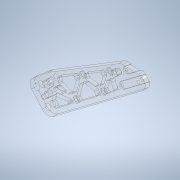
# Autodesk Inventor part: アーム アーム先端根本ポリカパーツ(ミラー)
Saved by Autodesk Inventor 2020.2 (Build 242310000, 310)
## iProperties
Created: 2020-05-02
Part Number: アーム アーム先端根本ポリカパーツ(ミラー)
Material: ポリカーボネート、クリア
Document SubType Name: Modeling
Designer: mozar
Density: 1.2 g/cm^3
Appearance: ポリカーボネート - クリア
Mass: 15.4398 g
Surface Area: 103.612 cm^2
Volume: 12.8665 cm^3
Author: mozar
Autodesk Inventor part; units mm, degrees
(part 1 of 2)
ref_plane "YZ Plane" through (0, 0, 0) normal (1, 0, 0) x (0, 1, 0)
ref_plane "XZ Plane" through (0, 0, 0) normal (0, 1, 0) x (-1, 0, 0)
ref_plane "XY Plane" through (0, 0, 0) normal (0, 0, 1) x (1, 0, 0)
sketch "スケッチ1" plane through (0, 0, 0) normal (0, 0, 1) x (1, 0, 0)
  circle A0 centre (-129.11052, 24.304119) radius 1.5
  circle A1 centre (-99.752673, 43.359743) radius 1.5
  circle A2 centre (-45.703772, 62.415368) radius 1.5
  circle A3 centre (-41.036979, 81.470992) radius 1.5
  circle A4 centre (-70.394826, 62.415368) radius 1.5
  circle A5 centre (-73.694174, 41.402576) radius 1.5
  circle A6 centre (-101.684575, 20.389785) radius 1.5
  circle A7 centre (-147.951739, 7.872185) radius 1.5
  line L0 (-23.449069, 99.142406) -> (-7.448842, 98.649717)
  arc A8 (-3.447491, 86.009971) -> (-7.448842, 98.649717) centre (-7.665058, 91.628045) ccw
  line L1 (-3.447491, 86.009971) -> (-131.660668, -10.24148)
  arc A9 (-141.440781, -10.106867) -> (-131.660668, -10.24148) centre (-136.463592, -3.843674) ccw
  line L2 (-141.440781, -10.106867) -> (-154.18878, 0.023621)
  arc A10 (-153.409815, 16.281111) -> (-154.18878, 0.023621) centre (-147.951739, 7.872185) ccw
  line L3 (-153.409815, 16.281111) -> (-27.490021, 98.013273)
  arc A11 (-23.449069, 99.142406) -> (-27.490021, 98.013273) centre (-23.665285, 92.120734) ccw
  circle A12 centre (-136.463592, -3.843674) radius 1.5
  circle A13 centre (-7.665058, 91.628045) radius 1.5
  circle A14 centre (-27.658202, 76.618908) radius 1.5
  circle A15 centre (-23.665285, 92.120734) radius 1.5
  circle A16 centre (-136.463592, -3.843674) radius 8
  circle A17 centre (-165.894632, -3.310235) radius 1.5
  circle A18 centre (-136.536785, 15.745389) radius 1.5
  circle A19 centre (-82.487883, 34.801014) radius 1.5
  circle A20 centre (-77.821091, 53.856638) radius 1.5
  circle A21 centre (-107.178938, 34.801014) radius 1.5
  circle A22 centre (-110.478285, 13.788222) radius 1.5
  circle A23 centre (-138.468687, -7.22457) radius 1.5
  circle A24 centre (-184.735851, -19.742169) radius 1.5
  circle A25 centre (-173.247704, -31.458028) radius 1.5
  circle A26 centre (-44.44917, 64.013691) radius 1.5
  circle A27 centre (-64.442314, 49.004554) radius 1.5
  circle A28 centre (-60.449397, 64.50638) radius 1.5
  line L4 (-64.274133, 70.398919) -> (-190.193926, -11.333243)
  arc A29 (-190.193926, -11.333243) -> (-190.972891, -27.590733) centre (-184.735851, -19.742169) ccw
  line L5 (-190.972891, -27.590733) -> (-178.224893, -37.721221)
  arc A30 (-178.224893, -37.721221) -> (-168.44478, -37.855834) centre (-173.247704, -31.458028) ccw
  line L6 (-168.44478, -37.855834) -> (-40.231602, 58.395617)
  arc A31 (-40.231602, 58.395617) -> (-44.232954, 71.035362) centre (-44.44917, 64.013691) ccw
  line L7 (-44.232954, 71.035362) -> (-60.233181, 71.528052)
  arc A32 (-60.233181, 71.528052) -> (-64.274133, 70.398919) centre (-60.449397, 64.50638) ccw
  circle A33 centre (-60.449397, 64.50638) radius 7.025
  circle A34 centre (-147.951739, 7.872185) radius 10.025
  line L8 (-153.154364, 16.44151) -> (-64.095126, 70.511318)
  point P0 (0, 0)
  point P1 (0, 0)
  point P2 (36.784112, 27.614354)
  constraints: 35 centre point, 20 point on circle, 18 end point, 2 coincident, 2 tangent, 54 other
extrude "押し出し1" add sketch "スケッチ1" against normal blind 5 contours A0 | A1 | A2 A26 | A4 | A5 | A6 | A34 L4 A10 | L1 A16 A34 L4 A33 L7 A31 | L4 A34 A16 A10 | L8 A32 L4 A34 | A9 A16 A34 | A34 A16 L2 | A32 A33 | A16 A34 | A18 | A19 | A20 | A21 | A22 | A23 picked at (-46.281723, 61.837664)
sketch "スケッチ2" plane through (0, 0, 0) normal (0, 0, 1) x (1, 0, 0)
  circle A0 centre (-64.442314, 49.004554) radius 1.5
  circle A1 centre (-44.44917, 64.013691) radius 1.5
  line L0 (-41.268818, 70.277554) -> (-66.303447, 51.483704)
  arc A2 (-37.546552, 65.319255) -> (-41.268818, 70.277554) centre (-44.44917, 64.013691) ccw
  line L1 (-62.581181, 46.525404) -> (-37.546552, 65.319255)
  arc A3 (-66.303447, 51.483704) -> (-62.581181, 46.525404) centre (-64.442314, 49.004554) ccw
  circle A4 centre (-60.449397, 64.50638) radius 1.5
  line L2 (-46.496021, 71.105048) -> (-56.416161, 71.410515)
  line L3 (-58.588264, 62.02723) -> (-46.496021, 71.105048)
  arc A5 (-62.310529, 66.98553) -> (-58.588264, 62.02723) centre (-60.449397, 64.50638) ccw
  line L4 (-56.416161, 71.410515) -> (-62.310529, 66.98553)
  point P0 (0, 0)
  point P1 (0, 0)
  constraints: 10 end point, 6 centre point, 6 point on circle, 25 other
extrude "押し出し2" cut sketch "スケッチ2" against normal blind 1
sketch "スケッチ3" plane through (0, 0, -5) normal (0, 0, -1) x (-1, 0, 0)
  line L0 (56.416161, 71.410515) -> (46.496021, 71.105048)
  line L1 (62.310529, 66.98553) -> (56.416161, 71.410515)
  arc A0 (58.588264, 62.02723) -> (62.310529, 66.98553) centre (60.449397, 64.50638) ccw
  line L2 (46.496021, 71.105048) -> (58.588264, 62.02723)
  circle A1 centre (60.449397, 64.50638) radius 1.5
  arc A2 (62.581181, 46.525404) -> (66.303447, 51.483704) centre (64.442314, 49.004554) ccw
  line L3 (37.546552, 65.319255) -> (62.581181, 46.525404)
  arc A3 (41.268818, 70.277554) -> (37.546552, 65.319255) centre (44.44917, 64.013691) ccw
  line L4 (66.303447, 51.483704) -> (41.268818, 70.277554)
  circle A4 centre (64.442314, 49.004554) radius 1.5
  circle A5 centre (44.44917, 64.013691) radius 1.5
  point P0 (0, 0)
extrude "押し出し3" cut sketch "スケッチ3" against normal blind 1
extrude "押し出し4" add sketch "スケッチ2" against normal blind 1
sketch "スケッチ4" plane through (0, 0, -5) normal (0, 0, -1) x (-1, 0, 0)
  line L0 (46.496021, 71.105048) -> (58.588264, 62.02723)
  arc A0 (58.588264, 62.02723) -> (62.310529, 66.98553) centre (60.449397, 64.50638) ccw
  line L1 (62.310529, 66.98553) -> (56.416161, 71.410515)
  line L2 (56.416161, 71.410515) -> (60.233181, 71.528052)
  arc A1 (64.095126, 70.511318) -> (60.233181, 71.528052) centre (60.449397, 64.50638) ccw
  line L3 (64.095126, 70.511318) -> (153.154364, 16.44151)
  arc A2 (154.18878, 0.023621) -> (153.154364, 16.44151) centre (147.951739, 7.872185) ccw
  line L4 (154.18878, 0.023621) -> (141.440781, -10.106867)
  arc A3 (131.660668, -10.24148) -> (141.440781, -10.106867) centre (136.463592, -3.843674) ccw
  line L5 (131.660668, -10.24148) -> (40.231602, 58.395617)
  arc A4 (37.546552, 65.319255) -> (40.231602, 58.395617) centre (44.44917, 64.013691) ccw
  line L6 (37.546552, 65.319255) -> (62.581181, 46.525404)
  arc A5 (62.581181, 46.525404) -> (66.303447, 51.483704) centre (64.442314, 49.004554) ccw
  line L7 (66.303447, 51.483704) -> (41.268818, 70.277554)
  arc A6 (44.232954, 71.035362) -> (41.268818, 70.277554) centre (44.44917, 64.013691) ccw
  line L8 (44.232954, 71.035362) -> (46.496021, 71.105048)
  circle A7 centre (136.463592, -3.843674) radius 1.5
  circle A8 centre (147.951739, 7.872185) radius 1.5
  circle A9 centre (147.951739, 7.872185) radius 3
  circle A10 centre (136.463592, -3.843674) radius 1.5
  circle A11 centre (136.463592, -3.843674) radius 3
  point P0 (0, 0)
  dimension "d8" = 6
  dimension "d9" = 6
  constraints: 2 centre point, 2 coincident
  measures "d8" diameter of A9
  measures "d9" diameter of A11
extrude "押し出し5" cut sketch "スケッチ4" against normal blind 1 contours A9 | A11
sketch "スケッチ5" plane through (0, 0, 0) normal (0, 0, 1) x (1, 0, 0)
  line L0 (-60.233181, 71.528052) -> (-44.232954, 71.035362)
  arc A0 (-40.231602, 58.395617) -> (-44.232954, 71.035362) centre (-44.44917, 64.013691) ccw
  line L1 (-40.231602, 58.395617) -> (-131.660668, -10.24148)
  arc A1 (-141.440781, -10.106867) -> (-131.660668, -10.24148) centre (-136.463592, -3.843674) ccw
  line L2 (-141.440781, -10.106867) -> (-154.18878, 0.023621)
  arc A2 (-153.154364, 16.44151) -> (-154.18878, 0.023621) centre (-147.951739, 7.872185) ccw
  line L3 (-153.154364, 16.44151) -> (-64.095126, 70.511318)
  arc A3 (-60.233181, 71.528052) -> (-64.095126, 70.511318) centre (-60.449397, 64.50638) ccw
  circle A4 centre (-147.951739, 7.872185) radius 1.5
  circle A5 centre (-136.463592, -3.843674) radius 1.5
  circle A6 centre (-60.449397, 64.50638) radius 1.5
  circle A7 centre (-64.442314, 49.004554) radius 1.5
  circle A8 centre (-44.44917, 64.013691) radius 1.5
  line L4 (-60.721853, 64.955147) -> (-149.781091, 10.885339)
  arc A9 (-149.781091, 10.885339) -> (-150.144813, 5.112465) centre (-147.951739, 7.872185) ccw
  line L5 (-150.144813, 5.112465) -> (-137.396815, -5.018022)
  arc A10 (-137.396815, -5.018022) -> (-135.563044, -5.043262) centre (-136.463592, -3.843674) ccw
  line L6 (-135.563044, -5.043262) -> (-44.133978, 63.593834)
  arc A11 (-44.133978, 63.593834) -> (-44.433011, 64.538442) centre (-44.44917, 64.013691) ccw
  line L7 (-44.433011, 64.538442) -> (-60.433238, 65.031131)
  arc A12 (-60.433238, 65.031131) -> (-60.721853, 64.955147) centre (-60.449397, 64.50638) ccw
  circle A13 centre (-77.811872, 54.579424) radius 3
  circle A14 centre (-84.115857, 33.578871) radius 3
  circle A15 centre (-105.248527, 37.922031) radius 3
  circle A16 centre (-112.106259, 12.566079) radius 3
  circle A17 centre (-132.685182, 21.264639) radius 3
  point P0 (0, 0)
  point P1 (0, 0)
  dimension "d12" = 6.5
  dimension "d13" = 6
  dimension "d14" = 6
  dimension "d15" = 6
  dimension "d16" = 6
  dimension "d17" = 6
  dimension "d18" = 104.18777
  dimension "d19" = 20
  dimension "d20" = 89.33084
  dimension "d21" = 25
  dimension "d22" = 35
  dimension "d23" = 20
  dimension "d24" = 64.19466
  dimension "d25" = 32.09733
  constraints: 18 centre point, 16 end point, 16 point on circle, 5 point on line, 7 other
  measures "d12" distance between parallel lines of L3 L4
  measures "d13" diameter of A13
  measures "d14" diameter of A14
  measures "d15" diameter of A15
  measures "d16" diameter of A16
  measures "d17" diameter of A17
  measures "d18" distance of L4.start L4.end
  measures "d19" distance of A3.centre A13.centre
  measures "d20" distance of A7.centre A5.centre
  measures "d21" distance of A7.centre A14.centre
  measures "d22" distance of A14.centre A16.centre
  measures "d23" distance of L4.end A17.centre
  measures "d24" distance of A13.centre A17.centre
  measures "d25" distance of A13.centre A15.centre
hole "穴1" at (-132.685182, 21.264639, 0) at (-105.248527, 37.922031, 0) at (-77.811872, 54.579424, 0) at (-84.115857, 33.578871, 0) at (-112.106259, 12.566079, 0) direction (0, 0, -1) diameter 3 depth 12 tip angle 118
sketch "スケッチ6" plane through (0, 0, -5) normal (0, 0, -1) x (-1, 0, 0)
  circle A0 centre (84.115857, 33.578871) radius 1.5
  circle A1 centre (105.248527, 37.922031) radius 1.5
  circle A2 centre (132.685182, 21.264639) radius 1.5
  circle A3 centre (77.811872, 54.579424) radius 1.5
  circle A4 centre (112.106259, 12.566079) radius 1.5
  circle A5 centre (136.463592, -3.843674) radius 3
  circle A6 centre (147.951739, 7.872185) radius 3
  line L0 (62.581181, 46.525404) -> (37.546552, 65.319255)
  arc A7 (37.546552, 65.319255) -> (40.231602, 58.395617) centre (44.44917, 64.013691) ccw
  line L1 (40.231602, 58.395617) -> (131.660668, -10.24148)
  arc A8 (131.660668, -10.24148) -> (141.440781, -10.106867) centre (136.463592, -3.843674) ccw
  line L2 (141.440781, -10.106867) -> (154.18878, 0.023621)
  arc A9 (154.18878, 0.023621) -> (153.154364, 16.44151) centre (147.951739, 7.872185) ccw
  line L3 (153.154364, 16.44151) -> (64.095126, 70.511318)
  arc A10 (64.095126, 70.511318) -> (60.233181, 71.528052) centre (60.449397, 64.50638) ccw
  line L4 (60.233181, 71.528052) -> (56.416161, 71.410515)
  line L5 (56.416161, 71.410515) -> (62.310529, 66.98553)
  arc A11 (58.588264, 62.02723) -> (62.310529, 66.98553) centre (60.449397, 64.50638) ccw
  line L6 (58.588264, 62.02723) -> (46.496021, 71.105048)
  line L7 (46.496021, 71.105048) -> (44.232954, 71.035362)
  arc A12 (44.232954, 71.035362) -> (41.268818, 70.277554) centre (44.44917, 64.013691) ccw
  line L8 (41.268818, 70.277554) -> (66.303447, 51.483704)
  arc A13 (62.581181, 46.525404) -> (66.303447, 51.483704) centre (64.442314, 49.004554) ccw
  circle A14 centre (77.811872, 54.579424) radius 3
  circle A15 centre (84.115857, 33.578871) radius 1.5
  circle A16 centre (84.115857, 33.578871) radius 3
  circle A17 centre (105.248527, 37.922031) radius 3
  circle A18 centre (112.106259, 12.566079) radius 1.5
  circle A19 centre (112.106259, 12.566079) radius 3
  circle A20 centre (132.685182, 21.264639) radius 1.5
  circle A21 centre (132.685182, 21.264639) radius 3
  point P0 (0, 0)
  dimension "d33" = 6
  dimension "d34" = 6
  dimension "d35" = 6
  dimension "d36" = 6
  dimension "d37" = 6
  constraints: 5 centre point, 5 coincident
  measures "d33" diameter of A14
  measures "d34" diameter of A16
  measures "d35" diameter of A17
  measures "d36" diameter of A19
  measures "d37" diameter of A21
extrude "押し出し6" cut sketch "スケッチ6" against normal blind 1 contours A0 | A1 | A2 | A3 | A4 | A14 | A16 | A17 | A19 | A21
sketch "スケッチ7" plane through (0, 0, 0) normal (0, 0, 1) x (1, 0, 0)
  circle A0 centre (-84.115857, 33.578871) radius 1.5
  circle A1 centre (-105.248527, 37.922031) radius 1.5
  circle A2 centre (-132.685182, 21.264639) radius 1.5
  circle A3 centre (-77.811872, 54.579424) radius 1.5
  circle A4 centre (-112.106259, 12.566079) radius 1.5
  circle A5 centre (-60.449397, 64.50638) radius 1.5
  circle A6 centre (-64.442314, 49.004554) radius 1.5
  circle A7 centre (-44.44917, 64.013691) radius 1.5
  line L0 (-44.232954, 71.035362) -> (-60.233181, 71.528052)
  arc A8 (-60.233181, 71.528052) -> (-64.095126, 70.511318) centre (-60.449397, 64.50638) ccw
  line L1 (-64.095126, 70.511318) -> (-153.154364, 16.44151)
  arc A9 (-153.154364, 16.44151) -> (-154.18878, 0.023621) centre (-147.951739, 7.872185) ccw
  line L2 (-154.18878, 0.023621) -> (-141.440781, -10.106867)
  arc A10 (-141.440781, -10.106867) -> (-131.660668, -10.24148) centre (-136.463592, -3.843674) ccw
  line L3 (-131.660668, -10.24148) -> (-40.231602, 58.395617)
  arc A11 (-40.231602, 58.395617) -> (-44.232954, 71.035362) centre (-44.44917, 64.013691) ccw
  circle A12 centre (-147.951739, 7.872185) radius 1.5
  circle A13 centre (-136.463592, -3.843674) radius 1.5
  circle A14 centre (-132.685182, 21.264639) radius 1.5
  circle A15 centre (-132.685182, 21.264639) radius 4.5
  circle A16 centre (-147.951739, 7.872185) radius 4.5
  circle A17 centre (-136.463592, -3.843674) radius 1.5
  circle A18 centre (-136.463592, -3.843674) radius 4.5
  line L4 (-151.164791, 4.721582) -> (-139.676644, -6.994276)
  line L5 (-132.013695, -4.513314) -> (-128.354238, 19.804531)
  line L6 (-135.652744, 24.647474) -> (-150.919302, 11.25502)
  point P0 (0, 0)
  dimension "d40" = 9
  dimension "d41" = 9
  dimension "d42" = 9
  constraints: 6 end point, 4 point on circle, 4 tangent, 3 coincident, 2 centre point, 5 other
  measures "d41" diameter of A16
  measures "d42" diameter of A18
sketch "スケッチ8" plane through (0, 0, -5) normal (0, 0, -1) x (-1, 0, 0)
  circle A0 centre (105.248527, 37.922031) radius 3
  circle A1 centre (132.685182, 21.264639) radius 3
  circle A2 centre (77.811872, 54.579424) radius 3
  circle A3 centre (112.106259, 12.566079) radius 3
  circle A4 centre (84.115857, 33.578871) radius 3
  circle A5 centre (136.463592, -3.843674) radius 3
  circle A6 centre (147.951739, 7.872185) radius 3
  line L0 (62.581181, 46.525404) -> (37.546552, 65.319255)
  arc A7 (37.546552, 65.319255) -> (40.231602, 58.395617) centre (44.44917, 64.013691) ccw
  line L1 (40.231602, 58.395617) -> (131.660668, -10.24148)
  arc A8 (131.660668, -10.24148) -> (141.440781, -10.106867) centre (136.463592, -3.843674) ccw
  line L2 (141.440781, -10.106867) -> (154.18878, 0.023621)
  arc A9 (154.18878, 0.023621) -> (153.154364, 16.44151) centre (147.951739, 7.872185) ccw
  line L3 (153.154364, 16.44151) -> (64.095126, 70.511318)
  arc A10 (64.095126, 70.511318) -> (60.233181, 71.528052) centre (60.449397, 64.50638) ccw
  line L4 (60.233181, 71.528052) -> (56.416161, 71.410515)
  line L5 (56.416161, 71.410515) -> (62.310529, 66.98553)
  arc A11 (58.588264, 62.02723) -> (62.310529, 66.98553) centre (60.449397, 64.50638) ccw
  line L6 (58.588264, 62.02723) -> (46.496021, 71.105048)
  line L7 (46.496021, 71.105048) -> (44.232954, 71.035362)
  arc A12 (44.232954, 71.035362) -> (41.268818, 70.277554) centre (44.44917, 64.013691) ccw
  line L8 (41.268818, 70.277554) -> (66.303447, 51.483704)
  arc A13 (62.581181, 46.525404) -> (66.303447, 51.483704) centre (64.442314, 49.004554) ccw
  circle A14 centre (136.463592, -3.843674) radius 4.5
  circle A15 centre (160.891456, -1.841844) radius 4.5
  line L9 (143.99842, -12.772755) -> (-26.359431, 7.016899)
  circle A16 centre (147.951739, 7.872185) radius 20.963209
  point P0 (0, 0)
  dimension "d43" = 9
  dimension "d44" = 9
  dimension "d45" = 24.26656
  dimension "d46" = 24.26656
  dimension "d47" = 30.27
  dimension "d48" = 41.92642
  constraints: 3 centre point, 2 coincident, 2 end point, 2 tangent
  measures "d43" diameter of A14
  measures "d44" diameter of A15
  measures "d45" distance from line of L1 A9.centre
  measures "d46" distance from line of L1 A15.centre
  measures "d47" angle of L9 L1
  measures "d48" diameter of A16
hole "穴2" at (-147.951739, 7.872185, 0) at (-132.685182, 21.264639, 0) at (-136.463592, -3.843674, 0) direction (0, 0, -1) diameter 6 depth 12 tip angle 118
sketch "スケッチ9" plane through (0, 0, -5) normal (0, 0, -1) x (-1, 0, 0)
  arc A0 (116.635058, 8.630348) -> (117.147544, 9.312551) centre (112.106259, 12.566079) ccw
  arc A1 (116.635058, 8.630348) -> (116.789492, 7.174667) centre (117.389857, 7.974392) ccw
  line L0 (116.789492, 7.174667) -> (129.297772, -2.215477)
  arc A2 (129.297772, -2.215477) -> (130.83606, -1.762597) centre (129.898137, -1.415751) ccw
  arc A3 (133.114093, 1.134364) -> (130.83606, -1.762597) centre (136.463592, -3.843674) ccw
  arc A4 (133.114093, 1.134364) -> (133.54471, 2.112846) centre (132.555844, 1.964037) ccw
  line L1 (133.54471, 2.112846) -> (132.792729, 7.109914)
  arc A5 (132.792729, 7.109914) -> (131.933702, 7.95264) centre (131.803863, 6.961105) ccw
  line L2 (131.933702, 7.95264) -> (118.117598, 9.761832)
  arc A6 (118.117598, 9.761832) -> (117.147544, 9.312551) centre (117.987758, 8.770297) ccw
  arc A7 (145.546046, 13.368787) -> (142.910454, 11.125713) centre (147.951739, 7.872185) ccw
  arc A8 (145.546046, 13.368787) -> (145.664062, 15.139683) centre (145.145097, 14.284888) ccw
  line L3 (145.664062, 15.139683) -> (139.431914, 18.923356)
  arc A9 (139.431914, 18.923356) -> (138.023268, 18.525143) centre (138.912949, 18.068561) ccw
  arc A10 (136.03468, 16.286601) -> (138.023268, 18.525143) centre (132.685182, 21.264639) ccw
  arc A11 (136.03468, 16.286601) -> (135.604064, 15.308119) centre (136.59293, 15.456928) ccw
  line L4 (135.604064, 15.308119) -> (136.075602, 12.174654)
  arc A12 (136.075602, 12.174654) -> (136.934628, 11.331928) centre (137.064468, 12.323463) ccw
  line L5 (136.934628, 11.331928) -> (141.9404, 10.676432)
  arc A13 (141.9404, 10.676432) -> (142.910454, 11.125713) centre (142.07024, 11.667967) ccw
  arc A14 (109.14609, 33.360343) -> (110.586613, 35.182536) centre (105.248527, 37.922031) ccw
  arc A15 (109.14609, 33.360343) -> (108.830366, 32.338983) centre (109.795684, 32.600062) ccw
  line L6 (108.830366, 32.338983) -> (112.38569, 19.19344)
  arc A16 (112.38569, 19.19344) -> (113.173186, 18.470456) centre (113.351007, 19.454519) ccw
  arc A17 (116.098395, 17.045236) -> (113.173186, 18.470456) centre (112.106259, 12.566079) ccw
  arc A18 (116.098395, 17.045236) -> (117.15309, 16.870668) centre (116.763751, 17.791763) ccw
  line L7 (117.15309, 16.870668) -> (126.080991, 20.644427)
  arc A19 (126.080991, 20.644427) -> (126.690727, 21.522538) centre (125.691651, 21.565521) ccw
  arc A20 (127.791923, 24.736817) -> (126.690727, 21.522538) centre (132.685182, 21.264639) ccw
  arc A21 (127.791923, 24.736817) -> (127.495344, 26.170308) centre (126.976379, 25.315513) ccw
  line L8 (127.495344, 26.170308) -> (111.995259, 35.580749)
  arc A22 (111.995259, 35.580749) -> (110.586613, 35.182536) centre (111.476294, 34.725953) ccw
  arc A23 (70.160292, 54.741689) -> (71.858452, 55.325612) centre (70.866216, 55.449977) ccw
  arc A24 (72.918613, 58.051601) -> (71.858452, 55.325612) centre (77.811872, 54.579424) ccw
  arc A25 (72.918613, 58.051601) -> (72.622035, 59.485093) centre (72.10307, 58.630298) ccw
  line L9 (72.622035, 59.485093) -> (69.229438, 61.544813)
  arc A26 (69.229438, 61.544813) -> (67.802662, 61.109398) centre (68.710473, 60.690017) ccw
  arc A27 (66.414464, 59.026602) -> (67.802662, 61.109398) centre (60.449397, 64.50638) ccw
  arc A28 (66.414464, 59.026602) -> (66.550527, 57.55036) centre (67.150892, 58.350086) ccw
  line L10 (66.550527, 57.55036) -> (69.305274, 55.482332)
  arc A29 (70.160292, 54.741689) -> (69.305274, 55.482332) centre (64.442314, 49.004554) ccw
  arc A30 (70.331118, 43.4429) -> (72.542276, 49.029257) centre (64.442314, 49.004554) ccw
  arc A31 (70.331118, 43.4429) -> (70.457765, 41.956551) centre (71.058131, 42.756277) ccw
  line L11 (70.457765, 41.956551) -> (77.631528, 36.571106)
  arc A32 (77.631528, 36.571106) -> (79.072459, 36.829123) centre (78.231893, 37.370832) ccw
  arc A33 (80.094406, 38.031727) -> (79.072459, 36.829123) centre (84.115857, 33.578871) ccw
  arc A34 (80.094406, 38.031727) -> (80.381942, 39.061377) centre (79.424164, 38.77387) ccw
  line L12 (80.381942, 39.061377) -> (77.714673, 47.946886)
  arc A35 (77.714673, 47.946886) -> (76.907606, 48.647957) centre (76.756895, 47.659379) ccw
  arc A36 (74.152214, 49.824752) -> (76.907606, 48.647957) centre (77.811872, 54.579424) ccw
  arc A37 (74.152214, 49.824752) -> (72.542276, 49.029257) centre (73.542271, 49.032306) ccw
  line L13 (123.324226, 13.114183) -> (130.745103, 12.142434)
  arc A38 (130.745103, 12.142434) -> (131.863809, 13.282778) centre (130.874943, 13.133969) ccw
  line L14 (131.863809, 13.282778) -> (131.6486, 14.712884)
  arc A39 (131.6486, 14.712884) -> (130.949084, 15.521298) centre (130.659734, 14.564075) ccw
  arc A40 (128.693046, 16.785482) -> (130.949084, 15.521298) centre (132.685182, 21.264639) ccw
  arc A41 (128.693046, 16.785482) -> (127.63835, 16.96005) centre (128.02769, 16.038956) ccw
  line L15 (127.63835, 16.96005) -> (123.064726, 15.026812)
  arc A42 (123.064726, 15.026812) -> (123.324226, 13.114183) centre (123.454066, 14.105718) ccw
  line L16 (99.456074, 34.689773) -> (90.713554, 32.89302)
  arc A43 (90.713554, 32.89302) -> (89.943579, 32.151404) centre (90.914866, 31.913493) ccw
  arc A44 (88.644656, 29.643139) -> (89.943579, 32.151404) centre (84.115857, 33.578871) ccw
  arc A45 (88.644656, 29.643139) -> (88.79909, 28.187458) centre (89.399456, 28.987184) ccw
  line L17 (88.79909, 28.187458) -> (105.621929, 15.558314)
  arc A46 (105.621929, 15.558314) -> (107.062861, 15.816331) centre (106.222295, 16.35804) ccw
  arc A47 (108.208695, 17.127767) -> (107.062861, 15.816331) centre (112.106259, 12.566079) ccw
  arc A48 (108.208695, 17.127767) -> (108.524419, 18.149127) centre (107.559102, 17.888049) ccw
  line L18 (108.524419, 18.149127) -> (104.969096, 31.29467)
  arc A49 (104.969096, 31.29467) -> (104.181599, 32.017655) centre (104.003778, 31.033592) ccw
  arc A50 (100.45612, 34.311929) -> (104.181599, 32.017655) centre (105.248527, 37.922031) ccw
  arc A51 (100.45612, 34.311929) -> (99.456074, 34.689773) centre (99.657386, 33.710245) ccw
  line L19 (100.058689, 42.827701) -> (84.558604, 52.238141)
  arc A52 (84.558604, 52.238141) -> (83.149958, 51.839928) centre (84.039639, 51.383346) ccw
  arc A53 (81.833323, 50.126568) -> (83.149958, 51.839928) centre (77.811872, 54.579424) ccw
  arc A54 (81.833323, 50.126568) -> (81.545787, 49.096917) centre (82.503565, 49.384425) ccw
  line L20 (81.545787, 49.096917) -> (84.213055, 40.211408)
  arc A55 (84.213055, 40.211408) -> (85.020123, 39.510338) centre (85.170834, 40.498916) ccw
  arc A56 (88.908264, 37.188973) -> (85.020123, 39.510338) centre (84.115857, 33.578871) ccw
  arc A57 (88.908264, 37.188973) -> (89.908309, 36.81113) centre (89.706998, 37.790657) ccw
  line L21 (89.908309, 36.81113) -> (98.650829, 38.607882)
  arc A58 (98.650829, 38.607882) -> (99.420805, 39.349498) centre (98.449518, 39.587409) ccw
  arc A59 (100.355268, 41.394209) -> (99.420805, 39.349498) centre (105.248527, 37.922031) ccw
  arc A60 (100.355268, 41.394209) -> (100.058689, 42.827701) centre (99.539724, 41.972905) ccw
  line L22 (141.421042, 6.710292) -> (138.123227, 7.142135)
  arc A61 (138.123227, 7.142135) -> (137.004522, 6.001791) centre (137.993388, 6.1506) ccw
  line L23 (137.004522, 6.001791) -> (137.500173, 2.708082)
  arc A62 (137.500173, 2.708082) -> (138.19969, 1.899667) centre (138.489039, 2.856891) ccw
  arc A63 (142.031716, -1.608501) -> (138.19969, 1.899667) centre (136.463592, -3.843674) ccw
  arc A64 (142.031716, -1.608501) -> (143.581885, -2.018871) centre (142.959736, -1.235972) ccw
  line L24 (143.581885, -2.018871) -> (146.594315, 0.375026)
  arc A65 (146.594315, 0.375026) -> (146.254963, 2.117105) centre (145.972167, 1.157925) ccw
  arc A66 (142.242708, 6.02639) -> (146.254963, 2.117105) centre (147.951739, 7.872185) ccw
  arc A67 (142.242708, 6.02639) -> (141.421042, 6.710292) centre (141.291203, 5.718757) ccw
  circle A68 centre (132.685182, 21.264639) radius 3
  circle A69 centre (105.248527, 37.922031) radius 3
  circle A70 centre (84.115857, 33.578871) radius 3
  circle A71 centre (77.811872, 54.579424) radius 3
  circle A72 centre (112.106259, 12.566079) radius 3
  circle A73 centre (136.463592, -3.843674) radius 3
  circle A74 centre (147.951739, 7.872185) radius 3
  line L25 (62.310529, 66.98553) -> (56.416161, 71.410515)
  line L26 (56.416161, 71.410515) -> (60.233181, 71.528052)
  arc A75 (64.095126, 70.511318) -> (60.233181, 71.528052) centre (60.449397, 64.50638) ccw
  line L27 (64.095126, 70.511318) -> (153.154364, 16.44151)
  arc A76 (154.18878, 0.023621) -> (153.154364, 16.44151) centre (147.951739, 7.872185) ccw
  line L28 (154.18878, 0.023621) -> (141.440781, -10.106867)
  arc A77 (131.660668, -10.24148) -> (141.440781, -10.106867) centre (136.463592, -3.843674) ccw
  line L29 (131.660668, -10.24148) -> (40.231602, 58.395617)
  arc A78 (37.546552, 65.319255) -> (40.231602, 58.395617) centre (44.44917, 64.013691) ccw
  line L30 (37.546552, 65.319255) -> (62.581181, 46.525404)
  arc A79 (62.581181, 46.525404) -> (66.303447, 51.483704) centre (64.442314, 49.004554) ccw
  line L31 (66.303447, 51.483704) -> (41.268818, 70.277554)
  arc A80 (44.232954, 71.035362) -> (41.268818, 70.277554) centre (44.44917, 64.013691) ccw
  line L32 (44.232954, 71.035362) -> (46.496021, 71.105048)
  line L33 (46.496021, 71.105048) -> (58.588264, 62.02723)
  arc A81 (58.588264, 62.02723) -> (62.310529, 66.98553) centre (60.449397, 64.50638) ccw
  point P0 (0, 0)
  point P1 (0, 0)
  constraints: 150 point on circle, 82 centre point, 68 end point, 307 other
extrude "押し出し7" cut sketch "スケッチ9" against normal blind 4 contours A0 A6 L2 A5 L1 A4 A3 A2 L0 A1 | A7 A13 L5 A12 L4 A11 A10 A9 L3 A8 | A14 A22 L8 A21 A20 A19 L7 A18 A17 A16 L6 A15 | A29 L10 A28 A27 A26 L9 A25 A24 A23 | A30 A37 A36 A35 L12 A34 A33 A32 L11 A31 | A42 L15 A41 A40 A39 L14 A38 L13 | A51 A50 A49 L18 A48 A47 A46 L17 A45 A44 A43 L16 | A60 A59 A58 L21 A57 A56 A55 L20 A54 A53 A52 L19 | A67 A66 A65 L24 A64 A63 A62 L23 A61 L22
sketch "スケッチ10" plane through (0, 0, -5) normal (0, 0, -1) x (-1, 0, 0)
  arc A0 (74.152214, 49.824752) -> (76.907606, 48.647957) centre (77.811872, 54.579424) ccw
  arc A1 (74.152214, 49.824752) -> (72.542276, 49.029257) centre (73.542271, 49.032306) ccw
  arc A2 (70.331118, 43.4429) -> (72.542276, 49.029257) centre (64.442314, 49.004554) ccw
  arc A3 (70.331118, 43.4429) -> (70.457765, 41.956551) centre (71.058131, 42.756277) ccw
  line L0 (70.457765, 41.956551) -> (77.631528, 36.571106)
  arc A4 (77.631528, 36.571106) -> (79.072459, 36.829123) centre (78.231893, 37.370832) ccw
  arc A5 (80.094406, 38.031727) -> (79.072459, 36.829123) centre (84.115857, 33.578871) ccw
  arc A6 (80.094406, 38.031727) -> (80.381942, 39.061377) centre (79.424164, 38.77387) ccw
  line L1 (80.381942, 39.061377) -> (77.714673, 47.946886)
  arc A7 (77.714673, 47.946886) -> (76.907606, 48.647957) centre (76.756895, 47.659379) ccw
  arc A8 (137.500173, 2.708082) -> (138.19969, 1.899667) centre (138.489039, 2.856891) ccw
  arc A9 (142.031716, -1.608501) -> (138.19969, 1.899667) centre (136.463592, -3.843674) ccw
  arc A10 (142.031716, -1.608501) -> (143.581885, -2.018871) centre (142.959736, -1.235972) ccw
  line L2 (143.581885, -2.018871) -> (146.594315, 0.375026)
  arc A11 (146.594315, 0.375026) -> (146.254963, 2.117105) centre (145.972167, 1.157925) ccw
  arc A12 (142.242708, 6.02639) -> (146.254963, 2.117105) centre (147.951739, 7.872185) ccw
  arc A13 (142.242708, 6.02639) -> (141.421042, 6.710292) centre (141.291203, 5.718757) ccw
  line L3 (141.421042, 6.710292) -> (138.123227, 7.142135)
  arc A14 (138.123227, 7.142135) -> (137.004522, 6.001791) centre (137.993388, 6.1506) ccw
  line L4 (137.004522, 6.001791) -> (137.500173, 2.708082)
  arc A15 (136.03468, 16.286601) -> (138.023268, 18.525143) centre (132.685182, 21.264639) ccw
  arc A16 (136.03468, 16.286601) -> (135.604064, 15.308119) centre (136.59293, 15.456928) ccw
  line L5 (135.604064, 15.308119) -> (136.075602, 12.174654)
  arc A17 (136.075602, 12.174654) -> (136.934628, 11.331928) centre (137.064468, 12.323463) ccw
  line L6 (136.934628, 11.331928) -> (141.9404, 10.676432)
  arc A18 (141.9404, 10.676432) -> (142.910454, 11.125713) centre (142.07024, 11.667967) ccw
  arc A19 (145.546046, 13.368787) -> (142.910454, 11.125713) centre (147.951739, 7.872185) ccw
  arc A20 (145.546046, 13.368787) -> (145.664062, 15.139683) centre (145.145097, 14.284888) ccw
  line L7 (145.664062, 15.139683) -> (139.431914, 18.923356)
  arc A21 (139.431914, 18.923356) -> (138.023268, 18.525143) centre (138.912949, 18.068561) ccw
  arc A22 (100.355268, 41.394209) -> (100.058689, 42.827701) centre (99.539724, 41.972905) ccw
  line L8 (100.058689, 42.827701) -> (84.558604, 52.238141)
  arc A23 (84.558604, 52.238141) -> (83.149958, 51.839928) centre (84.039639, 51.383346) ccw
  arc A24 (81.833323, 50.126568) -> (83.149958, 51.839928) centre (77.811872, 54.579424) ccw
  arc A25 (81.833323, 50.126568) -> (81.545787, 49.096917) centre (82.503565, 49.384425) ccw
  line L9 (81.545787, 49.096917) -> (84.213055, 40.211408)
  arc A26 (84.213055, 40.211408) -> (85.020123, 39.510338) centre (85.170834, 40.498916) ccw
  arc A27 (88.908264, 37.188973) -> (85.020123, 39.510338) centre (84.115857, 33.578871) ccw
  arc A28 (88.908264, 37.188973) -> (89.908309, 36.81113) centre (89.706998, 37.790657) ccw
  line L10 (89.908309, 36.81113) -> (98.650829, 38.607882)
  arc A29 (98.650829, 38.607882) -> (99.420805, 39.349498) centre (98.449518, 39.587409) ccw
  arc A30 (100.355268, 41.394209) -> (99.420805, 39.349498) centre (105.248527, 37.922031) ccw
  arc A31 (70.160292, 54.741689) -> (71.858452, 55.325612) centre (70.866216, 55.449977) ccw
  arc A32 (72.918613, 58.051601) -> (71.858452, 55.325612) centre (77.811872, 54.579424) ccw
  arc A33 (72.918613, 58.051601) -> (72.622035, 59.485093) centre (72.10307, 58.630298) ccw
  line L11 (72.622035, 59.485093) -> (69.229438, 61.544813)
  arc A34 (69.229438, 61.544813) -> (67.802662, 61.109398) centre (68.710473, 60.690017) ccw
  arc A35 (66.414464, 59.026602) -> (67.802662, 61.109398) centre (60.449397, 64.50638) ccw
  arc A36 (66.414464, 59.026602) -> (66.550527, 57.55036) centre (67.150892, 58.350086) ccw
  line L12 (66.550527, 57.55036) -> (69.305274, 55.482332)
  arc A37 (70.160292, 54.741689) -> (69.305274, 55.482332) centre (64.442314, 49.004554) ccw
  arc A38 (127.791923, 24.736817) -> (126.690727, 21.522538) centre (132.685182, 21.264639) ccw
  arc A39 (127.791923, 24.736817) -> (127.495344, 26.170308) centre (126.976379, 25.315513) ccw
  line L13 (127.495344, 26.170308) -> (111.995259, 35.580749)
  arc A40 (111.995259, 35.580749) -> (110.586613, 35.182536) centre (111.476294, 34.725953) ccw
  arc A41 (109.14609, 33.360343) -> (110.586613, 35.182536) centre (105.248527, 37.922031) ccw
  arc A42 (109.14609, 33.360343) -> (108.830366, 32.338983) centre (109.795684, 32.600062) ccw
  line L14 (108.830366, 32.338983) -> (112.38569, 19.19344)
  arc A43 (112.38569, 19.19344) -> (113.173186, 18.470456) centre (113.351007, 19.454519) ccw
  arc A44 (116.098395, 17.045236) -> (113.173186, 18.470456) centre (112.106259, 12.566079) ccw
  arc A45 (116.098395, 17.045236) -> (117.15309, 16.870668) centre (116.763751, 17.791763) ccw
  line L15 (117.15309, 16.870668) -> (126.080991, 20.644427)
  arc A46 (126.080991, 20.644427) -> (126.690727, 21.522538) centre (125.691651, 21.565521) ccw
  line L16 (123.324226, 13.114183) -> (130.745103, 12.142434)
  arc A47 (130.745103, 12.142434) -> (131.863809, 13.282778) centre (130.874943, 13.133969) ccw
  line L17 (131.863809, 13.282778) -> (131.6486, 14.712884)
  arc A48 (131.6486, 14.712884) -> (130.949084, 15.521298) centre (130.659734, 14.564075) ccw
  arc A49 (128.693046, 16.785482) -> (130.949084, 15.521298) centre (132.685182, 21.264639) ccw
  arc A50 (128.693046, 16.785482) -> (127.63835, 16.96005) centre (128.02769, 16.038956) ccw
  line L18 (127.63835, 16.96005) -> (123.064726, 15.026812)
  arc A51 (123.064726, 15.026812) -> (123.324226, 13.114183) centre (123.454066, 14.105718) ccw
  arc A52 (88.644656, 29.643139) -> (88.79909, 28.187458) centre (89.399456, 28.987184) ccw
  line L19 (88.79909, 28.187458) -> (105.621929, 15.558314)
  arc A53 (105.621929, 15.558314) -> (107.062861, 15.816331) centre (106.222295, 16.35804) ccw
  arc A54 (108.208695, 17.127767) -> (107.062861, 15.816331) centre (112.106259, 12.566079) ccw
  arc A55 (108.208695, 17.127767) -> (108.524419, 18.149127) centre (107.559102, 17.888049) ccw
  line L20 (108.524419, 18.149127) -> (104.969096, 31.29467)
  arc A56 (104.969096, 31.29467) -> (104.181599, 32.017655) centre (104.003778, 31.033592) ccw
  arc A57 (100.45612, 34.311929) -> (104.181599, 32.017655) centre (105.248527, 37.922031) ccw
  arc A58 (100.45612, 34.311929) -> (99.456074, 34.689773) centre (99.657386, 33.710245) ccw
  line L21 (99.456074, 34.689773) -> (90.713554, 32.89302)
  arc A59 (90.713554, 32.89302) -> (89.943579, 32.151404) centre (90.914866, 31.913493) ccw
  arc A60 (88.644656, 29.643139) -> (89.943579, 32.151404) centre (84.115857, 33.578871) ccw
  arc A61 (133.114093, 1.134364) -> (133.54471, 2.112846) centre (132.555844, 1.964037) ccw
  line L22 (133.54471, 2.112846) -> (132.792729, 7.109914)
  arc A62 (132.792729, 7.109914) -> (131.933702, 7.95264) centre (131.803863, 6.961105) ccw
  line L23 (131.933702, 7.95264) -> (118.117598, 9.761832)
  arc A63 (118.117598, 9.761832) -> (117.147544, 9.312551) centre (117.987758, 8.770297) ccw
  arc A64 (116.635058, 8.630348) -> (117.147544, 9.312551) centre (112.106259, 12.566079) ccw
  arc A65 (116.635058, 8.630348) -> (116.789492, 7.174667) centre (117.389857, 7.974392) ccw
  line L24 (116.789492, 7.174667) -> (129.297772, -2.215477)
  arc A66 (129.297772, -2.215477) -> (130.83606, -1.762597) centre (129.898137, -1.415751) ccw
  arc A67 (133.114093, 1.134364) -> (130.83606, -1.762597) centre (136.463592, -3.843674) ccw
  circle A68 centre (105.248527, 37.922031) radius 3
  circle A69 centre (132.685182, 21.264639) radius 3
  circle A70 centre (77.811872, 54.579424) radius 3
  circle A71 centre (112.106259, 12.566079) radius 3
  circle A72 centre (84.115857, 33.578871) radius 3
  circle A73 centre (136.463592, -3.843674) radius 3
  circle A74 centre (147.951739, 7.872185) radius 3
  line L25 (46.496021, 71.105048) -> (58.588264, 62.02723)
  arc A75 (58.588264, 62.02723) -> (62.310529, 66.98553) centre (60.449397, 64.50638) ccw
  line L26 (62.310529, 66.98553) -> (56.416161, 71.410515)
  line L27 (56.416161, 71.410515) -> (60.233181, 71.528052)
  arc A76 (64.095126, 70.511318) -> (60.233181, 71.528052) centre (60.449397, 64.50638) ccw
  line L28 (64.095126, 70.511318) -> (153.154364, 16.44151)
  arc A77 (154.18878, 0.023621) -> (153.154364, 16.44151) centre (147.951739, 7.872185) ccw
  line L29 (154.18878, 0.023621) -> (141.440781, -10.106867)
  arc A78 (131.660668, -10.24148) -> (141.440781, -10.106867) centre (136.463592, -3.843674) ccw
  line L30 (131.660668, -10.24148) -> (40.231602, 58.395617)
  arc A79 (37.546552, 65.319255) -> (40.231602, 58.395617) centre (44.44917, 64.013691) ccw
  line L31 (37.546552, 65.319255) -> (62.581181, 46.525404)
  arc A80 (62.581181, 46.525404) -> (66.303447, 51.483704) centre (64.442314, 49.004554) ccw
  line L32 (66.303447, 51.483704) -> (41.268818, 70.277554)
  arc A81 (44.232954, 71.035362) -> (41.268818, 70.277554) centre (44.44917, 64.013691) ccw
  line L33 (44.232954, 71.035362) -> (46.496021, 71.105048)
  circle A82 centre (136.463592, -3.843674) radius 8
  circle A83 centre (147.951739, 7.872185) radius 7
  circle A84 centre (132.685182, 21.264639) radius 6.5
  line L34 (136.850058, 26.255011) -> (152.436991, 13.246431)
  line L35 (153.239213, 3.284961) -> (142.506418, -9.086216)
  circle A85 centre (112.106259, 12.566079) radius 1.5
  arc A86 (116.098395, 17.045236) -> (113.173186, 18.470456) centre (112.106259, 12.566079) ccw
  circle A87 centre (112.106259, 12.566079) radius 6.5
  line L36 (131.660668, -10.24148) -> (108.203883, 7.367862)
  line L37 (40.231602, 58.395617) -> (131.660668, -10.24148)
  point P0 (0, 0)
  point P1 (136.058454, 26.82081)
  point P2 (108.203883, 7.367862)
  point P3 (131.660668, -10.24148)
  point P4 (131.660668, -10.24148)
  dimension "d58" = 5
  dimension "d59" = 4
  constraints: 6 end point, 4 point on circle, 4 tangent, 2 centre point, 1 coincident, 10 other
  measures "d58" radial gap between concentric circles of A73 A82
  measures "d59" radial gap between concentric circles of A74 A83
extrude "押し出し10" cut sketch "スケッチ10" against normal blind 10 contours L35 A83 L34 A84 L28 A77 L29 A82
sketch "スケッチ12" plane through (0, 0, -5) normal (0, 0, -1) x (-1, 0, 0)
  arc A0 (74.152214, 49.824752) -> (76.907606, 48.647957) centre (77.811872, 54.579424) ccw
  arc A1 (74.152214, 49.824752) -> (72.542276, 49.029257) centre (73.542271, 49.032306) ccw
  arc A2 (70.331118, 43.4429) -> (72.542276, 49.029257) centre (64.442314, 49.004554) ccw
  arc A3 (70.331118, 43.4429) -> (70.457765, 41.956551) centre (71.058131, 42.756277) ccw
  line L0 (70.457765, 41.956551) -> (77.631528, 36.571106)
  arc A4 (77.631528, 36.571106) -> (79.072459, 36.829123) centre (78.231893, 37.370832) ccw
  arc A5 (80.094406, 38.031727) -> (79.072459, 36.829123) centre (84.115857, 33.578871) ccw
  arc A6 (80.094406, 38.031727) -> (80.381942, 39.061377) centre (79.424164, 38.77387) ccw
  line L1 (80.381942, 39.061377) -> (77.714673, 47.946886)
  arc A7 (77.714673, 47.946886) -> (76.907606, 48.647957) centre (76.756895, 47.659379) ccw
  arc A8 (137.500173, 2.708082) -> (138.19969, 1.899667) centre (138.489039, 2.856891) ccw
  arc A9 (142.031716, -1.608501) -> (138.19969, 1.899667) centre (136.463592, -3.843674) ccw
  arc A10 (142.031716, -1.608501) -> (143.581885, -2.018871) centre (142.959736, -1.235972) ccw
  line L2 (143.581885, -2.018871) -> (146.594315, 0.375026)
  arc A11 (146.594315, 0.375026) -> (146.254963, 2.117105) centre (145.972167, 1.157925) ccw
  arc A12 (142.242708, 6.02639) -> (146.254963, 2.117105) centre (147.951739, 7.872185) ccw
  arc A13 (142.242708, 6.02639) -> (141.421042, 6.710292) centre (141.291203, 5.718757) ccw
  line L3 (141.421042, 6.710292) -> (138.123227, 7.142135)
  arc A14 (138.123227, 7.142135) -> (137.004522, 6.001791) centre (137.993388, 6.1506) ccw
  line L4 (137.004522, 6.001791) -> (137.500173, 2.708082)
  arc A15 (136.03468, 16.286601) -> (138.023268, 18.525143) centre (132.685182, 21.264639) ccw
  arc A16 (136.03468, 16.286601) -> (135.604064, 15.308119) centre (136.59293, 15.456928) ccw
  line L5 (135.604064, 15.308119) -> (136.075602, 12.174654)
  arc A17 (136.075602, 12.174654) -> (136.934628, 11.331928) centre (137.064468, 12.323463) ccw
  line L6 (136.934628, 11.331928) -> (141.9404, 10.676432)
  arc A18 (141.9404, 10.676432) -> (142.910454, 11.125713) centre (142.07024, 11.667967) ccw
  arc A19 (145.546046, 13.368787) -> (142.910454, 11.125713) centre (147.951739, 7.872185) ccw
  arc A20 (145.546046, 13.368787) -> (145.664062, 15.139683) centre (145.145097, 14.284888) ccw
  line L7 (145.664062, 15.139683) -> (139.431914, 18.923356)
  arc A21 (139.431914, 18.923356) -> (138.023268, 18.525143) centre (138.912949, 18.068561) ccw
  arc A22 (100.355268, 41.394209) -> (100.058689, 42.827701) centre (99.539724, 41.972905) ccw
  line L8 (100.058689, 42.827701) -> (84.558604, 52.238141)
  arc A23 (84.558604, 52.238141) -> (83.149958, 51.839928) centre (84.039639, 51.383346) ccw
  arc A24 (81.833323, 50.126568) -> (83.149958, 51.839928) centre (77.811872, 54.579424) ccw
  arc A25 (81.833323, 50.126568) -> (81.545787, 49.096917) centre (82.503565, 49.384425) ccw
  line L9 (81.545787, 49.096917) -> (84.213055, 40.211408)
  arc A26 (84.213055, 40.211408) -> (85.020123, 39.510338) centre (85.170834, 40.498916) ccw
  arc A27 (88.908264, 37.188973) -> (85.020123, 39.510338) centre (84.115857, 33.578871) ccw
  arc A28 (88.908264, 37.188973) -> (89.908309, 36.81113) centre (89.706998, 37.790657) ccw
  line L10 (89.908309, 36.81113) -> (98.650829, 38.607882)
  arc A29 (98.650829, 38.607882) -> (99.420805, 39.349498) centre (98.449518, 39.587409) ccw
  arc A30 (100.355268, 41.394209) -> (99.420805, 39.349498) centre (105.248527, 37.922031) ccw
  arc A31 (70.160292, 54.741689) -> (71.858452, 55.325612) centre (70.866216, 55.449977) ccw
  arc A32 (72.918613, 58.051601) -> (71.858452, 55.325612) centre (77.811872, 54.579424) ccw
  arc A33 (72.918613, 58.051601) -> (72.622035, 59.485093) centre (72.10307, 58.630298) ccw
  line L11 (72.622035, 59.485093) -> (69.229438, 61.544813)
  arc A34 (69.229438, 61.544813) -> (67.802662, 61.109398) centre (68.710473, 60.690017) ccw
  arc A35 (66.414464, 59.026602) -> (67.802662, 61.109398) centre (60.449397, 64.50638) ccw
  arc A36 (66.414464, 59.026602) -> (66.550527, 57.55036) centre (67.150892, 58.350086) ccw
  line L12 (66.550527, 57.55036) -> (69.305274, 55.482332)
  arc A37 (70.160292, 54.741689) -> (69.305274, 55.482332) centre (64.442314, 49.004554) ccw
  arc A38 (127.791923, 24.736817) -> (126.690727, 21.522538) centre (132.685182, 21.264639) ccw
  arc A39 (127.791923, 24.736817) -> (127.495344, 26.170308) centre (126.976379, 25.315513) ccw
  line L13 (127.495344, 26.170308) -> (111.995259, 35.580749)
  arc A40 (111.995259, 35.580749) -> (110.586613, 35.182536) centre (111.476294, 34.725953) ccw
  arc A41 (109.14609, 33.360343) -> (110.586613, 35.182536) centre (105.248527, 37.922031) ccw
  arc A42 (109.14609, 33.360343) -> (108.830366, 32.338983) centre (109.795684, 32.600062) ccw
  line L14 (108.830366, 32.338983) -> (112.38569, 19.19344)
  arc A43 (112.38569, 19.19344) -> (113.173186, 18.470456) centre (113.351007, 19.454519) ccw
  arc A44 (116.098395, 17.045236) -> (113.173186, 18.470456) centre (112.106259, 12.566079) ccw
  arc A45 (116.098395, 17.045236) -> (117.15309, 16.870668) centre (116.763751, 17.791763) ccw
  line L15 (117.15309, 16.870668) -> (126.080991, 20.644427)
  arc A46 (126.080991, 20.644427) -> (126.690727, 21.522538) centre (125.691651, 21.565521) ccw
  line L16 (123.324226, 13.114183) -> (130.745103, 12.142434)
  arc A47 (130.745103, 12.142434) -> (131.863809, 13.282778) centre (130.874943, 13.133969) ccw
  line L17 (131.863809, 13.282778) -> (131.6486, 14.712884)
  arc A48 (131.6486, 14.712884) -> (130.949084, 15.521298) centre (130.659734, 14.564075) ccw
  arc A49 (128.693046, 16.785482) -> (130.949084, 15.521298) centre (132.685182, 21.264639) ccw
  arc A50 (128.693046, 16.785482) -> (127.63835, 16.96005) centre (128.02769, 16.038956) ccw
  line L18 (127.63835, 16.96005) -> (123.064726, 15.026812)
  arc A51 (123.064726, 15.026812) -> (123.324226, 13.114183) centre (123.454066, 14.105718) ccw
  arc A52 (88.644656, 29.643139) -> (88.79909, 28.187458) centre (89.399456, 28.987184) ccw
  line L19 (88.79909, 28.187458) -> (105.621929, 15.558314)
  arc A53 (105.621929, 15.558314) -> (107.062861, 15.816331) centre (106.222295, 16.35804) ccw
  arc A54 (108.208695, 17.127767) -> (107.062861, 15.816331) centre (112.106259, 12.566079) ccw
  arc A55 (108.208695, 17.127767) -> (108.524419, 18.149127) centre (107.559102, 17.888049) ccw
  line L20 (108.524419, 18.149127) -> (104.969096, 31.29467)
  arc A56 (104.969096, 31.29467) -> (104.181599, 32.017655) centre (104.003778, 31.033592) ccw
  arc A57 (100.45612, 34.311929) -> (104.181599, 32.017655) centre (105.248527, 37.922031) ccw
  arc A58 (100.45612, 34.311929) -> (99.456074, 34.689773) centre (99.657386, 33.710245) ccw
  line L21 (99.456074, 34.689773) -> (90.713554, 32.89302)
  arc A59 (90.713554, 32.89302) -> (89.943579, 32.151404) centre (90.914866, 31.913493) ccw
  arc A60 (88.644656, 29.643139) -> (89.943579, 32.151404) centre (84.115857, 33.578871) ccw
  arc A61 (133.114093, 1.134364) -> (133.54471, 2.112846) centre (132.555844, 1.964037) ccw
  line L22 (133.54471, 2.112846) -> (132.792729, 7.109914)
  arc A62 (132.792729, 7.109914) -> (131.933702, 7.95264) centre (131.803863, 6.961105) ccw
  line L23 (131.933702, 7.95264) -> (118.117598, 9.761832)
  arc A63 (118.117598, 9.761832) -> (117.147544, 9.312551) centre (117.987758, 8.770297) ccw
  arc A64 (116.635058, 8.630348) -> (117.147544, 9.312551) centre (112.106259, 12.566079) ccw
  arc A65 (116.635058, 8.630348) -> (116.789492, 7.174667) centre (117.389857, 7.974392) ccw
  line L24 (116.789492, 7.174667) -> (129.297772, -2.215477)
  arc A66 (129.297772, -2.215477) -> (130.83606, -1.762597) centre (129.898137, -1.415751) ccw
  arc A67 (133.114093, 1.134364) -> (130.83606, -1.762597) centre (136.463592, -3.843674) ccw
  circle A68 centre (105.248527, 37.922031) radius 3
  circle A69 centre (132.685182, 21.264639) radius 3
  circle A70 centre (77.811872, 54.579424) radius 3
  circle A71 centre (112.106259, 12.566079) radius 3
  circle A72 centre (84.115857, 33.578871) radius 3
  circle A73 centre (136.463592, -3.843674) radius 3
  circle A74 centre (147.951739, 7.872185) radius 3
  line L25 (46.496021, 71.105048) -> (58.588264, 62.02723)
  arc A75 (58.588264, 62.02723) -> (62.310529, 66.98553) centre (60.449397, 64.50638) ccw
  line L26 (62.310529, 66.98553) -> (56.416161, 71.410515)
  line L27 (56.416161, 71.410515) -> (60.233181, 71.528052)
  arc A76 (64.095126, 70.511318) -> (60.233181, 71.528052) centre (60.449397, 64.50638) ccw
  line L28 (64.095126, 70.511318) -> (136.058454, 26.82081)
  arc A77 (136.850058, 26.255011) -> (136.058454, 26.82081) centre (132.685182, 21.264639) ccw
  line L29 (136.850058, 26.255011) -> (152.436991, 13.246431)
  arc A78 (153.239213, 3.284961) -> (152.436991, 13.246431) centre (147.951739, 7.872185) ccw
  line L30 (153.239213, 3.284961) -> (142.506418, -9.086216)
  arc A79 (131.660668, -10.24148) -> (142.506418, -9.086216) centre (136.463592, -3.843674) ccw
  line L31 (131.660668, -10.24148) -> (40.231602, 58.395617)
  arc A80 (37.546552, 65.319255) -> (40.231602, 58.395617) centre (44.44917, 64.013691) ccw
  line L32 (37.546552, 65.319255) -> (62.581181, 46.525404)
  arc A81 (62.581181, 46.525404) -> (66.303447, 51.483704) centre (64.442314, 49.004554) ccw
  line L33 (66.303447, 51.483704) -> (41.268818, 70.277554)
  arc A82 (44.232954, 71.035362) -> (41.268818, 70.277554) centre (44.44917, 64.013691) ccw
  line L34 (44.232954, 71.035362) -> (46.496021, 71.105048)
  arc A83 (153.239213, 3.284961) -> (152.436991, 13.246431) centre (147.951739, 7.872185) ccw
  circle A84 centre (147.951739, 7.872185) radius 7
  circle A85 centre (132.685182, 21.264639) radius 6.5
  point P0 (0, 0)
  constraints: 2 coincident, 6 other